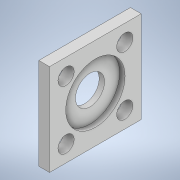
# Autodesk Inventor part: BearingSpacer
Saved by Autodesk Inventor 2020 (Build 240168000, 168)
## iProperties
Created: 2020-09-22
Part Number: BearingSpacer
Material: Generic
Document SubType Name: Modeling
Designer: tdmp4
Density: 1 g/cm^3
Appearance: Default
Author: tdmp4
Autodesk Inventor part; units mm, degrees
ref_plane "YZ Plane" through (0, 0, 0) normal (1, 0, 0) x (0, 1, 0)
ref_plane "XZ Plane" through (0, 0, 0) normal (0, 1, 0) x (-1, 0, 0)
ref_plane "XY Plane" through (0, 0, 0) normal (0, 0, 1) x (1, 0, 0)
sketch "Sketch1" plane through (0, 0, 0) normal (1, 0, 0) x (0, 1, 0)
  line L0 (0, 0) -> (21.59, 0)
  line L1 (21.59, 0) -> (21.59, -21.59)
  line L2 (21.59, -21.59) -> (0, -21.59)
  line L3 (0, -21.59) -> (0, 0)
  circle A0 centre (17.7098, -3.8802) radius 1.905
  circle A1 centre (17.7098, -17.7098) radius 1.905
  circle A2 centre (3.8802, -17.7098) radius 1.905
  circle A3 centre (3.8802, -3.8802) radius 1.905
  dimension "d0" = 21.59
  dimension "d1" = 21.59
  dimension "d3" = 3.81
  dimension "d4" = 3.81
  dimension "d5" = 3.81
  dimension "d6" = 3.81
  constraints: 8 end point, 4 centre point, 2 parallel, 1 horizontal, 1 perpendicular
  measures "d0" distance of L1.end L2.end
  measures "d1" distance of L0.end L1.end
  measures "d3" diameter of A0
  measures "d4" diameter of A1
  measures "d5" diameter of A2
  measures "d6" diameter of A3
extrude "Extrusion1" add sketch "Sketch1" along normal blind 2.54
sketch "Sketch2" plane through (2.54, 0, 0) normal (1, 0, 0) x (0, 0, -1)
  line L0 (21.59, 0) -> (21.59, 21.59) projected
  line L1 (21.59, 21.59) -> (0, 21.59) projected
  line L2 (0, 21.59) -> (0, 0) projected
  circle A0 centre (10.795, 10.795) radius 6.985
  dimension "d9" = 13.97
  constraints: 1 centre point
  measures "d9" diameter of A0
extrude "Extrusion2" cut sketch "Sketch2" against normal blind 1.27
sketch "Sketch3" plane through (1.27, 10.795, -10.795) normal (1, 0, 0) x (0, 0, -1)
  circle A0 centre (0, 0) radius 3.429
  point P0 (-10.795, -10.795)
  dimension "d12" = 6.858
  constraints: 1 centre point
  measures "d12" diameter of A0
extrude "Extrusion3" cut sketch "Sketch3" against normal blind 24.13
body "Solid1"
